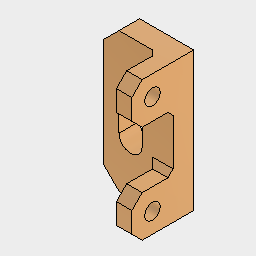
Y End Stop Bracket (Autodesk Fusion 360 design; units mm, degrees)
Autodesk Fusion 360 part; units mm, degrees
sketch "Sketch1" plane through (-37, -14, -9.5) normal (0, -1, 0) x (1, 0, 0)
  line L0 (42.5, 33.5) -> (38.5, 29.5)
  line L1 (38.5, 29.5) -> (38.5, 12)
  line L2 (38.5, 12) -> (23.5, 12)
  line L3 (23.5, 12) -> (23.5, 9.5)
  line L4 (23.5, 9.5) -> (54.5, 9.5)
  line L5 (54.5, 9.5) -> (54.5, 29.5)
  line L6 (54.5, 29.5) -> (50.5, 33.5)
  line L7 (50.5, 33.5) -> (42.5, 33.5)
  circle A0 centre (46.5, 23.5) radius 2.75 construction
  line L8 (51.75, 10) -> (41.25, 10)
  line L9 (41.25, 10) -> (41.25, 37)
  line L10 (41.25, 37) -> (51.75, 37)
  line L11 (51.75, 37) -> (51.75, 10)
  line L12 (51.75, 10) -> (41.25, 37) construction
  line L13 (41.25, 10) -> (51.75, 37) construction
  line L14 (51.75, 37) -> (54.75, 37)
  line L15 (54.75, 37) -> (54.75, 10)
  line L16 (54.75, 10) -> (51.75, 10)
  line L17 (51.75, 10) -> (51.75, 37)
  line L18 (46.5, 23.5) -> (54.75, 23.5) construction
  line L19 (54.75, 29) -> (51.75, 29)
  line L20 (51.75, 18) -> (54.75, 18)
  line L21 (54.5, 22.5) -> (61.5, 22.5)
  line L22 (61.5, 24.5) -> (54.5, 24.5)
  line L23 (54.5, 24.5) -> (54.5, 22.5)
  line L24 (44.25, 27.25) -> (44.25, 19.75)
  arc A1 (44.25, 19.75) -> (48.75, 19.75) centre (46.5, 19.75) ccw
  line L25 (48.75, 19.75) -> (48.75, 27.25)
  arc A2 (48.75, 27.25) -> (44.25, 27.25) centre (46.5, 27.25) ccw
  line L26 (46.5, 29.5) -> (46.5, 17.5) construction
  line L27 (61.5, 22.5) -> (61.5, 24.5)
  point P0 (46.5, 23.5)
  dimension "d4158" = 27
  dimension "d4161" = 3
  dimension "d4162" = 11
  dimension "d4195" = 4.5
  dimension "d4197" = 12
  dimension "d4207" = 3
  measures "d4158" distance of L8.end L9.end
  measures "d4161" distance of L10.end L14.end
  measures "d4162" distance of L19.end L20.start
  measures "d4195" diameter of A1
  measures "d4197" distance of L26.start L26.end
  measures "d4207" distance of L9 L24
extrude "Extrude1" add sketch "Sketch1" along normal blind 4 contours L0 L6 L7 L8 L9 L11 L17 | L0 L6 L7 L9 L10 L11 L17 | L5 L11 L17 L19 L20 L23 | L5 L15 L19 L22 | L5 L15 L20 L21 | L5 L15 L21 L22 L23
extrude "Extrude2" add sketch "Sketch1" along normal blind 12 contours L5 L6 L11 L14 L15 L17 L19 | L5 L6 L11 L17 L19 | L5 L11 L16 L17 L20 | L5 L15 L16 L20
sketch "Sketch2" plane through (14.75, 0, 0) normal (-1, 0, 0) x (0, -1, 0)
  line L0 (18, 27.5) -> (18, 19.5)
  line L1 (18, 19.5) -> (26, 19.5)
  line L2 (26, 19.5) -> (26, 27.5)
  line L3 (26, 27.5) -> (18, 27.5)
  line L4 (18, 8.5) -> (18, 0.5)
  line L5 (18, 0.5) -> (26, 0.5)
  line L6 (26, 0.5) -> (26, 8.5)
  line L7 (26, 8.5) -> (18, 8.5)
  line L8 (18, 27.5) -> (18, 0.5)
  line L9 (18, 14) -> (22, 14) construction
  line L10 (22, 23.625) -> (22, 4.375) construction
  point P0 (22, 27.5)
  dimension "d4168" = 19.25
  measures "d4168" distance of L10.start L10.end
hole "Hole1" at (14.75, -22, 23.625) at (14.75, -22, 4.375) direction (1, 0, 0) diameter 3 depth 5 tip angle 118
chamfer "Chamfer2" distance 1 angle 45 4 edges at (14.75, -18, 23.5) (14.75, -18, 4.5) (16.25, -18, 8.5) (16.25, -18, 19.5)
chamfer "Chamfer3" distance 3 angle 45 2 edges at (4.25, -16, 27.5) (4.25, -16, 0.5)
chamfer "Chamfer4" distance 2 angle 45 4 edges at (16.25, -26, 27.5) (16.25, -26, 19.5) (16.25, -26, 8.5) (16.25, -26, 0.5)
named bodies: "Y End Stop Bracket"
